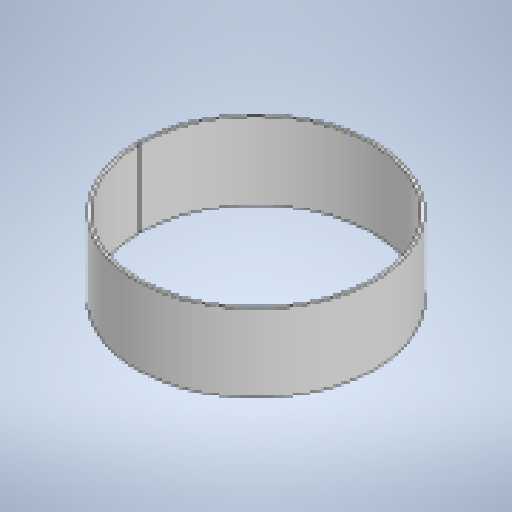
# Autodesk Inventor part: ANP 14031 accses hatch tube
Saved by Autodesk Inventor 2025 (Build 290162010, 162A)
## iProperties
Created: 2025-02-12
Part Number: ANP 14031 accses hatch tube
Material: Steel
Document SubType Name: Sheet Metal
Designer: pokla
Density: 7.85 g/cm^3
Flat Pattern Width: 17 cm
Flat Pattern Length: 163.719 cm
Flat Pattern Area: 2783.23 cm^2
Sheet Metal Rule: Default_mm
Sheet Metal Width: 170,000 mm
Sheet Metal Length: 1637,195 mm
Sheet Metal Area: 278323,068 mm^2
Appearance: Default
Mass: 13177.4 g
Surface Area: 5813.4 cm^2
Volume: 1678.65 cm^3
Author: pokla
Autodesk Inventor part; units mm, degrees
ref_plane "YZ Plane" through (0, 0, 0) normal (1, 0, 0) x (0, 1, 0)
ref_plane "XZ Plane" through (0, 0, 0) normal (0, 1, 0) x (-1, 0, 0)
ref_plane "XY Plane" through (0, 0, 0) normal (0, 0, 1) x (1, 0, 0)
sketch "Sketch1" plane through (0, 0, 0) normal (0, 1, 0) x (-1, 0, 0)
  line L0 (258, 120) -> (258, 0)
  line L1 (258, 0) -> (264, 0)
  line L2 (0, 0) -> (0, 109.131)
  line L3 (258, 120) -> (264, 120)
  line L4 (264, 0) -> (264, 120)
  line L5 (264, 0) -> (258, 0)
  line L6 (258, 0) -> (258, -50)
  line L7 (258, -50) -> (264, -50)
  line L8 (264, -50) -> (264, 0)
  point P0 (261, 0)
  point P1 (264, 0)
  point P2 (258, 0)
  point P3 (258, 0)
  dimension "d3" = 6
  dimension "d5" = 120
  dimension "d7" = 6
  dimension "d8" = 50
  dimension "d12" = 528
  constraints: 18 end point, 2 horizontal, 2 midpoint, 2 parallel, 2 perpendicular, 2 vertical, 1 horizontal alignment
  measures "d3" distance of L0.end L1.end
  measures "d5" distance between parallel lines of L1 L3
  measures "d7" distance of L6.end L7.end
  measures "d8" distance of L7.end L5.start
  measures "d12" diameter of L4 L2
revolve "Revolution1" add sketch "Sketch1" angle 359.9 about axis through (0, 0, 0) along (0, 0, 1)
sketch "Sketch2" plane through (0, 0, 0) normal (0, 1, 0) x (-1, 0, 0)
  circle A0 centre (0, -706) radius 706
  point P0 (0, 0)
  dimension "d9" = 1412
  constraints: 2 vertical alignment, 2 other
extrude "Extrusion1" [suppressed]
equation "\"d5\" = Accsess_hatch_lenght"
equation "\"d7\" = d3"
equation "\"BendRadius\" = Thickness"
equation "\"BendReliefWidth\" = Thickness"
equation "\"BendReliefDepth\" = 0.5 * Thickness"
equation "\"CornerReliefSize\" = 4 * Thickness"
equation "\"MinimumRemnant\" = 2 * Thickness"
equation "\"TransitionRadius\" = BendRadius"
equation "\"JacobiRadiusSize\" = BendRadius"
equation "\"GapSize\" = Thickness"
equation "\"Accsess_hatch_lenght\" = 120"
equation "\"Thickness\" = 6"
body "Solid1"
